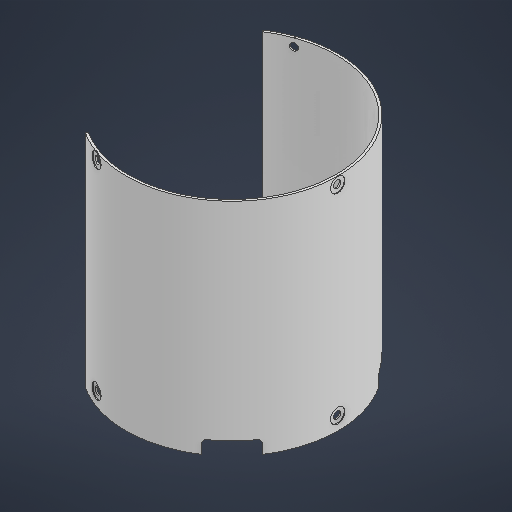
# Autodesk Inventor part: Abdeckung_Chamber
Saved by Autodesk Inventor 2027 (Build 310192060, 192F)
## iProperties
Created: 2026-08-01
Part Number: Abdeckung_Chamber
Material: Generic
Document SubType Name: Modeling
Designer: kw
Density: 1 g/cm^3
Appearance: Default
Author: kw
Autodesk Inventor part; units mm, degrees
ref_plane "XZ Plane" through (0, 0, 0) normal (0, 1, 0) x (-1, 0, 0)
ref_plane "XY Plane" through (0, 0, 0) normal (0, 0, 1) x (1, 0, 0)
sketch "Sketch1" plane through (0, 0, 0) normal (0, 1, 0) x (-1, 0, 0)
  circle A0 centre (0, 0) radius 47
  circle A1 centre (0, 0) radius 48
  line L0 (0, 0) -> (26.255, 40.183)
  line L1 (0, 0) -> (48, 0) construction
  line L2 (0, 0) -> (26.255, -40.183)
  line L3 (0, 0) -> (48, 0) construction
  point P0 (0, 48)
  point P1 (25.708, -39.3459)
  point P2 (25.708, 39.3459)
  dimension "d0" = 94
  dimension "d1" = 1
  dimension "d5" = 56.84
  dimension "d6" = 56.84
  constraints: 8 end point, 4 point on circle, 2 centre point, 2 equal length, 2 horizontal, 1 coincident
  measures "d0" diameter of A0
  measures "d1" radial gap between concentric circles of A0 A1
  measures "d5" angle of L1 L0
  measures "d6" angle of L2 L3
extrude "Extrusion1" add sketch "Sketch1" along normal blind 100 contours A0 L2 A1 L0 picked at (-47.1693, 0)
ref_plane "Work Plane1" through (48, 0, 0) normal (1, 0, 0) x (0, 1, 0)
sketch "Sketch2" plane through (48, 0, 0) normal (1, 0, 0) x (0, 1, 0)
  line L0 (100, -48) -> (100, 48) projected
  line L1 (100, 0) -> (96.5, 0)
  point P0 (0, 0)
  point P1 (6, 0)
  point P2 (100, 40.183)
  point P3 (100, -40.183)
  dimension "d26" = 3.5
  constraints: 2 end point, 1 horizontal, 1 midpoint
  measures "d26" distance of L1.start L1.end
hole "Hole1" at (48, 6, 0) at (48, 96.5, 0) direction (-1, 0, 0) diameter 3.2 depth 2 counterbore diameter 6.5 counterbore depth 0.4 clearance for "Socket Head Cap Screw ISO 4762" size "M3" standard "ISO"
pattern_circular "Circular Pattern1" count 3 over 220 about axis through (0, 0, 0) along (0, 1, 0) of "Hole1" both ways yes
sketch "Sketch3" plane through (0, 0, 0) normal (0, -1, 0) x (1, 0, 0)
  line L0 (0, 0) -> (26.255, -40.183)
  arc A0 (-26.255, -40.183) -> (-26.255, 40.183) centre (0, 0) ccw projected
  line L1 (0, 0) -> (48, 0) construction
  line L2 (0, 0) -> (26.255, 40.183)
  line L3 (0, 0) -> (48, 0) construction
  line L4 (0, 0) -> (40.183, -26.255)
  line L5 (0, 0) -> (48, 0) construction
  line L6 (0, 0) -> (40.183, 26.255)
  line L7 (0, 0) -> (48, 0) construction
  dimension "d20" = 56.84
  dimension "d21" = 56.84
  dimension "d22" = 33.16
  dimension "d23" = 33.16
  constraints: 16 end point, 4 equal length, 4 horizontal, 4 point on circle
  measures "d20" angle of L0 L1
  measures "d21" angle of L3 L2
  measures "d22" angle of L4 L5
  measures "d23" angle of L7 L6
extrude "Extrusion2" cut sketch "Sketch3" against normal blind 6 contours L4 A0 L0 | L2 A0 L6
fillet "Fillet1" radius 2 4 edges at (25.9815, 6, 39.7645) (39.7645, 6, 25.9815) (25.9815, 6, -39.7645) (39.7645, 6, -25.9815)
equation "\"d5\" = d6"
equation "\"d21\" = d20"
equation "\"d23\" = d22"
body "Solid1"
